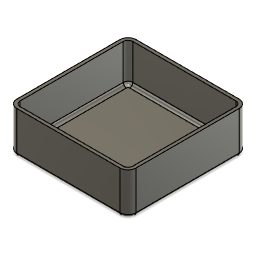
Parametric Box (Autodesk Fusion 360 design; units mm, degrees)
Autodesk Fusion 360 part; units mm, degrees
note: some values were not read from the file. Set by a fixed rule: which face or edge a step refers to.
sketch "Basis" plane through (0, 0, 0) normal (0, 1, 0) x (1, 0, 0)
  line L0 (5, 0) -> (69, 0)
  line L1 (74, 5) -> (74, 69)
  line L2 (69, 74) -> (5, 74)
  line L3 (0, 69) -> (0, 5)
  arc A0 (69, 0) -> (74, 5) centre (69, 5) ccw
  arc A1 (0, 5) -> (5, 0) centre (5, 5) ccw
  arc A2 (74, 69) -> (69, 74) centre (69, 69) ccw
  arc A3 (5, 74) -> (0, 69) centre (5, 69) ccw
  point P0 (74, 0)
  point P1 (0, 74)
  dimension "d1" = 74
  dimension "d2" = 74
  dimension "d18" = 5
  dimension "d19" = 5
  dimension "d20" = 5
  dimension "d21" = 5
  constraint horizontal L0
  constraint vertical L1
  constraint horizontal L2
  constraint vertical L3
  constraint coincident P0 L0
  constraint coincident P0 L1
  constraint tangent L0 A0
  constraint tangent L1 A0
  constraint coincident origin L0
  constraint coincident origin L3
  constraint tangent L0 A1
  constraint tangent L3 A1
  constraint tangent L1 A2
  constraint tangent L2 A2
  constraint coincident P1 L2
  constraint coincident P1 L3
  constraint tangent L2 A3
  constraint tangent L3 A3
  measures "d1" distance of origin P0
  measures "d2" distance of origin P1
  measures "d18" radius of A0
  measures "d19" radius of A1
  measures "d20" radius of A2
  measures "d21" radius of A3
extrude "Extrude1" add sketch "Basis" along normal blind 26
shell "Shell1" thickness 2 removed faces 1 at (26.3333, 26, -49.3333)
fillet "Fillet8" radius 2 8 edges at (72, 2, -37) (71.1213, 2, -71.1213) (37, 2, -72) (2.8787, 2, -71.1213) (2, 2, -37) (2.8787, 2, -2.8787) (37, 2, -2) (71.1213, 2, -2.8787)
fillet "Fillet9" radius 2 8 edges at (74, 0, -37) (72.5355, 0, -72.5355) (37, 0, -74) (1.4645, 0, -72.5355) (0, 0, -37) (1.4645, 0, -1.4645) (37, 0, 0) (72.5355, 0, -1.4645)
sketch "Label" plane through (72, 0, 0) normal (-1, 0, 0) x (0, 0, 1)
  line L0 (-69, 4) -> (-5, 4)
  line L1 (-69, 26) -> (-69, 4)
  line L2 (-2, 26) -> (-9.1154, 12.795)
  line L3 (-2, 26) -> (-2, 4)
  line L4 (-2, 4) -> (-9.1154, 12.795)
  line L5 (0, 2) -> (0, 26)
  point P0 (-2, 0)
  dimension "d28" = 15
  dimension "d31" = 2
  dimension "d35" = 26
  dimension "d38" = 22
  constraint parallel L3 L5
  measures "d28" distance of L2.start L2.end
  measures "d31" distance of L3 L5
  measures "d35" distance of L2.start P0
  measures "d38" distance of L2.start L3.end
extrude "Extrude2" add sketch "Label" along normal up to surface (70 mm away)
fillet "Fillet10" radius 1 1 edges at (37, 12.795, -9.1154)
equation "d1 = Width"
equation "d2 = Length"
equation "d3 = Height"
equation "Width = SegmentLen * 1"
equation "Height = SegmentHeight * 1"
equation "Length = SegmentLen * 1"
equation "d35 = Height"
equation "SegmentLen = 74 mm"
equation "SegmentHeight = 26 mm"
named bodies: "Box"
